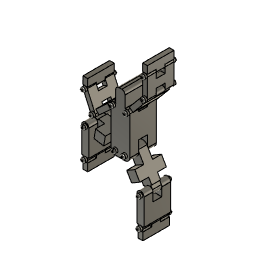
climber v7 (Autodesk Fusion 360 design; units mm, degrees)
Autodesk Fusion 360 part; units mm, degrees
sketch "Sketch1" plane through (0, 0, 0) normal (0, 1, 0) x (1, 0, 0) in component "climberTorso&Head"
  line L0 (1.4167, 0) -> (4.25, 0)
  line L1 (5.6667, -1.4167) -> (5.6667, -12.8917)
  line L2 (4.9583, -13.6) -> (0.7083, -13.6)
  line L3 (0, -12.8917) -> (0, -1.4167)
  circle A0 centre (0.7083, -12.8917) radius 0.25
  circle A1 centre (4.9583, -12.8917) radius 0.25
  circle A2 centre (1.4167, -1.4167) radius 0.25
  circle A3 centre (4.25, -1.4167) radius 0.25
  line L4 (1.4167, -13.6) -> (4.25, -13.6)
  line L5 (4.25, -13.6) -> (4.25, -17.1333)
  line L6 (3.25, -18.1333) -> (2.4167, -18.1333)
  line L7 (1.4167, -17.1333) -> (1.4167, -13.6)
  arc A4 (1.4167, -17.1333) -> (2.4167, -18.1333) centre (2.4167, -17.1333) ccw
  arc A5 (3.25, -18.1333) -> (4.25, -17.1333) centre (3.25, -17.1333) ccw
  line L8 (4.9583, -12.8917) -> (0.7083, -12.8917) construction
  line L9 (1.4167, -13.6) -> (1.4167, -12.8917) construction
  line L10 (1.4167, -12.8917) -> (1.4167, -13.6)
  line L11 (4.25, -12.8917) -> (4.25, -13.6)
  line L12 (4.9583, -12.1833) -> (5.6667, -12.1833)
  arc A6 (4.9583, -13.6) -> (5.6667, -12.8917) centre (4.9583, -12.8917) ccw
  arc A7 (4.9583, -12.1833) -> (4.25, -12.8917) centre (4.9583, -12.8917) ccw
  arc A8 (1.4167, -12.8917) -> (1.2092, -12.3908) centre (0.7083, -12.8917) ccw
  arc A9 (0, -12.8917) -> (0.7083, -13.6) centre (0.7083, -12.8917) ccw
  line L13 (0.7083, -12.8917) -> (0.7083, -12.1833) construction
  line L14 (4.9583, -12.8917) -> (4.9583, -12.1833) construction
  line L15 (4.25, -1.4167) -> (4.25, -2.8333) construction
  line L16 (1.4167, -1.4167) -> (1.4167, -2.8333) construction
  line L17 (1.4167, -2.8333) -> (0, -2.8333) construction
  line L18 (1.4167, -2.8333) -> (0, -2.8333)
  arc A10 (5.6667, -1.4167) -> (4.25, 0) centre (4.25, -1.4167) ccw
  arc A11 (2.8333, -1.4167) -> (3.2483, -2.4184) centre (4.25, -1.4167) ccw
  arc A12 (1.4167, 0) -> (0, -1.4167) centre (1.4167, -1.4167) ccw
  arc A13 (2.4184, -2.4184) -> (2.8333, -1.4167) centre (1.4167, -1.4167) ccw
  line L19 (1.2092, -12.3908) -> (0, -11.1816)
  line L20 (0.7083, -12.8917) -> (1.2092, -12.3908) construction
  line L21 (1.2092, -12.3908) -> (0, -11.1816)
  line L22 (1.2092, -12.3908) -> (0, -11.1816)
  circle A14 centre (1.4167, -1.4167) radius 1.4167 construction
  circle A15 centre (4.25, -1.4167) radius 1.4167 construction
  line L23 (1.4167, -1.4167) -> (2.4184, -2.4184) construction
  line L24 (4.25, -1.4167) -> (3.2483, -2.4184) construction
  line L25 (3.2483, -2.4184) -> (5.6667, -4.8368) construction
  line L26 (2.4184, -2.4184) -> (0, -4.8368) construction
  line L27 (3.2483, -2.4184) -> (5.6667, -4.8368)
  line L28 (2.4184, -2.4184) -> (0, -4.8368)
  point P0 (5.6667, 0)
  point P1 (0, -13.6)
  point P2 (1.4167, -18.1333)
  dimension "d69" = 5.6667
  dimension "d70" = 13.6
  dimension "d71" = 0.5
  dimension "d73" = 0.7083
  dimension "d75" = 0.7083
  dimension "d88" = 2.8333
  dimension "d89" = 4.5333
  dimension "d90" = 1
  dimension "d91" = 1
  dimension "d118" = 0.7083
  dimension "d145" = 1.4167
  dimension "d146" = 1.4167
  dimension "d149" = 0.7083
  dimension "d151" = 0.7083
  dimension "d152" = 0.7083
  dimension "d303" = 1.4167
  dimension "d304" = 1.4167
  dimension "d305" = 1.4167
  dimension "d306" = 2.8333
  dimension "d307" = 2.8333
  dimension "d308" = 1.4167
  dimension "d358" = 90
  constraint horizontal L0
  constraint vertical L1
  constraint horizontal L2
  constraint vertical L3
  constraint equal A1 A3
  constraint equal A0 A1
  constraint equal A0 A2
  constraint horizontal A2.centre A3.centre
  constraint horizontal A0.centre A1.centre
  constraint coincident P1 L2
  constraint coincident P1 L3
  constraint coincident origin L0
  constraint coincident origin L3
  constraint coincident P0 L0
  constraint coincident P0 L1
  constraint horizontal L4
  constraint vertical L5
  constraint horizontal L6
  constraint vertical L7
  constraint coincident P2 L6
  constraint coincident P2 L7
  constraint tangent L6 A4
  constraint tangent L7 A4
  constraint tangent L5 A5
  constraint tangent L6 A5
  constraint concentric A0 A8
  constraint coincident L3.start A8
  constraint concentric A1 A6
  constraint coincident A1.centre L8.start
  constraint coincident A0.centre L8.end
  constraint coincident L8 L9.end
  constraint tangent L9 A8
  constraint perpendicular L4 L10
  constraint coincident L8 L11.start
  constraint perpendicular L2 L11
  constraint coincident L12.start A6
  constraint perpendicular L1 L12
  constraint concentric A6 A7
  constraint concentric A8 A9
  constraint perpendicular L12 L14
  constraint concentric A2 A12
  constraint concentric A3 A10
  constraint coincident A3.centre L15.start
  constraint vertical L15
  constraint coincident A2.centre L16.start
  constraint coincident L16.end A12
  constraint vertical L16
  constraint coincident L3 L17.end
  constraint tangent L17 A12
  constraint perpendicular L3 L18
  constraint concentric A10 A11
  constraint concentric A12 A13
  constraint coincident L3 L19.end
  constraint perpendicular L19 L20
  constraint concentric A13 A14
  constraint concentric A10 A15
  constraint perpendicular L23 L24
  constraint coincident L1 L25.end
  constraint tangent A11 L25
  constraint perpendicular L24 L25
  constraint coincident L3 L26.end
  constraint tangent A15 L27
  measures "d69" distance of origin P0
  measures "d70" distance of origin P1
  measures "d71" diameter of A0
  measures "d73" distance of L2 A0.centre
  measures "d75" distance of L1 A1.centre
  measures "d88" distance of L4.start L4.end
  measures "d89" distance of L4.start P2
  measures "d90" radius of A4
  measures "d91" radius of A5
  measures "d118" distance of L3 A0.centre
  measures "d145" diameter of A8
  measures "d146" diameter of A6
  measures "d149" distance of L9.end L4.start
  measures "d151" distance of L11.start L4.end
  measures "d152" distance of L12.start L12.end
  measures "d303" distance of L3 A2.centre
  measures "d304" distance of L1 A3.centre
  measures "d305" distance of L0 A3.centre
  measures "d306" diameter of A12
  measures "d307" diameter of A10
  measures "d308" distance of L16.end L17.end
  measures "d358" angle of L25 L26
extrude "Extrude2" add sketch "Sketch1" along normal mid plane 8 makes body 1 in component "climberTorso&Head"
sketch "Sketch2" plane through (0, 0, 0) normal (0, 1, 0) x (1, 0, 0) in component "climberUpperArms"
  line L0 (1.4167, 2.1237) -> (1.4167, -6.0929)
  line L1 (0, -6.0929) -> (0, 2.1237)
  circle A0 centre (0.7083, -6.0929) radius 0.25
  circle A1 centre (0.7083, 2.1237) radius 0.25
  circle A2 centre (0.7083, -6.0929) radius 0.7083
  circle A3 centre (0.7083, 2.1237) radius 0.7083
  line L2 (0.7083, -6.0929) -> (0.7083, 2.1237) construction
  line L3 (0.7083, -5.3846) -> (0, -5.3846) construction
  line L4 (0.7083, -6.8013) -> (0.7083, 2.8321) construction
  line L5 (0.7083, -6.0929) -> (1.2092, -5.5921) construction
  line L6 (0.7083, -6.0929) -> (1.4167, -6.0929) construction
  line L7 (0.7083, -5.3846) -> (1.7101, -5.3846) construction
  line L8 (1.2092, -5.5921) -> (0, -4.3829) construction
  line L9 (1.2092, -5.5921) -> (-0.5009, -5.5921) construction
  line L10 (0, -4.3829) -> (1.4167, -4.3829)
  line L11 (0.7083, 2.1237) -> (1.2092, 1.6229) construction
  line L12 (0.7083, 2.1237) -> (1.4167, 2.1237) construction
  line L13 (1.2092, 1.6229) -> (0, 0.4137) construction
  line L14 (1.2092, 1.6229) -> (2.9193, 1.6229) construction
  line L15 (0, 0.4137) -> (1.4167, 0.4137)
  dimension "d106" = 0.5
  dimension "d108" = 0.7083
  dimension "d119" = 1.4167
  dimension "d120" = 1.4167
  dimension "d121" = 1.4167
  dimension "d132" = 0.7083
  dimension "d336" = 9.6333
  dimension "d341" = 45
  dimension "d342" = 0.7083
  dimension "d344" = 45
  dimension "d480" = 45
  dimension "d481" = 135
  constraint vertical L0
  constraint vertical L1
  constraint equal A0 A1
  constraint vertical A0.centre A1.centre
  constraint concentric A0 A2
  constraint concentric A1 A3
  constraint coincident A3 L1.end
  constraint coincident A3 L0.start
  constraint coincident A2 L1.start
  constraint coincident A2 L0.end
  constraint coincident A0.centre A2.centre
  constraint coincident A1.centre A3.centre
  constraint coincident L2 L3.start
  constraint coincident A2 L3.start
  constraint perpendicular L1 L3
  constraint coincident A2 L4.start
  constraint coincident A3 L4.end
  constraint horizontal L6
  constraint horizontal L7
  constraint horizontal L9
  constraint coincident L1 L8.end
  constraint coincident L0 L10.end
  constraint perpendicular L0 L10
  constraint horizontal L12
  constraint coincident A3 L11.end
  constraint horizontal L14
  constraint coincident L1 L13.end
  constraint coincident L0 L15.end
  constraint perpendicular L0 L15
  measures "d106" diameter of A0
  measures "d108" distance of L1 A0.centre
  measures "d119" diameter of A2
  measures "d120" diameter of A3
  measures "d121" distance of L0 L1
  measures "d132" distance of L3.start L3.end
  measures "d336" distance of L4.start L4.end
  measures "d341" angle of L5 L6
  measures "d342" distance of A0.centre L5.end
  measures "d344" angle of L8 L9
  measures "d480" angle of L11 L12
  measures "d481" angle of L13 L14
extrude "Extrude3" add sketch "Sketch2" along normal mid plane 2.6667 separate body contours A3 | L0 L1 A3 L15 | L0 L1 A2 L10 | A2 makes body 2 at (1.4158, 0.4444, 6.1282) makes body 3 at (0.1657, -0.4444, -2.579) in component "climberUpperArms"
extrude "Extrude2'" add sketch "Sketch2" along normal mid plane 8 separate body contours L0 L1 L10 L15 makes body 4 in component "climberUpperArms"
extrude "Extrude3'" cut sketch "Sketch1" along normal mid plane 2.6667 contours L0 L1 L3 A10 A11 A12 A13 L27 L28 | L1 L2 L11 L12 A6 A7 | L2 L3 L10 A8 A9 L19 L21 L22 | A0 | A1 | A2 | A3 bodies 1 in component "climberTorso&Head"
sketch "Sketch1 (2)" plane through (0, 0, 0) normal (0, 1, 0) x (1, 0, 0) in component "climberLowerArms"
  line L0 (3.9167, -0.375) -> (3.9167, -6.325)
  line L1 (2.5, -6.325) -> (2.5, -0.375)
  circle A0 centre (3.2083, -6.325) radius 0.25
  circle A1 centre (3.2083, -0.375) radius 0.25
  line L2 (3.2083, -6.325) -> (3.2083, -0.375) construction
  arc A2 (2.5, -6.325) -> (3.9167, -6.325) centre (3.2083, -6.325) ccw
  arc A3 (3.9167, -0.375) -> (2.5, -0.375) centre (3.2083, -0.375) ccw
  line L3 (3.2083, -6.325) -> (3.2083, -7.0333) construction
  line L4 (3.2083, -0.375) -> (3.2083, 0.3333) construction
  circle A4 centre (3.2083, -6.325) radius 0.7083 construction
  circle A5 centre (3.2083, -0.375) radius 0.7083 construction
  line L5 (3.2083, -6.325) -> (3.7092, -5.8241) construction
  line L6 (3.2083, -6.325) -> (3.9167, -6.325) construction
  line L7 (3.7092, -5.8241) -> (2.5, -4.6149) construction
  line L8 (2.5, -4.6149) -> (3.9167, -4.6149)
  line L9 (3.2083, -0.375) -> (3.7092, -0.8759) construction
  line L10 (3.2083, -0.375) -> (3.9167, -0.375) construction
  line L11 (3.7092, -0.8759) -> (2.5, -2.0851) construction
  line L12 (2.5, -2.0851) -> (3.9167, -2.0851)
  dimension "d186" = 0.5
  dimension "d188" = 0.7083
  dimension "d191" = 1.4167
  dimension "d192" = 1.4167
  dimension "d200" = 1.4167
  dimension "d201" = 7.3667
  dimension "d267" = 0
  dimension "d268" = 0
  dimension "d269" = 0
  dimension "d270" = 0
  dimension "d337" = 1.4167
  dimension "d338" = 1.4167
  dimension "d482" = 45
  dimension "d483" = 90
  dimension "d484" = 45
  dimension "d485" = 45
  dimension "d486" = 90
  dimension "d487" = 45
  constraint vertical L0
  constraint vertical L1
  constraint equal A0 A1
  constraint vertical A0.centre A1.centre
  constraint concentric A0 A2
  constraint concentric A1 A3
  constraint coincident A0.centre L2.start
  constraint coincident A1.centre L2.end
  constraint midpoint A2 L3.end
  constraint parallel L2 L3
  constraint midpoint A3 L4.end
  constraint parallel L2 L4
  constraint concentric A0 A4
  constraint concentric A1 A5
  constraint horizontal L6
  constraint coincident A4 L5.end
  constraint coincident L1 L7.end
  constraint coincident L0 L8.end
  constraint horizontal L10
  constraint coincident A5 L9.end
  constraint coincident L1 L11.end
  constraint coincident L0 L12.end
  measures "d186" diameter of A0
  measures "d188" distance of L1 A0.centre
  measures "d191" diameter of A2
  measures "d192" diameter of A3
  measures "d200" distance of L0 L1
  measures "d201" distance of L3.end L4.end
  measures "d337" diameter of A4
  measures "d338" diameter of A5
  measures "d482" angle of L5 L6
  measures "d483" angle of L5 L7
  measures "d484" angle of L7 L8
  measures "d485" angle of L9 L10
  measures "d486" angle of L9 L11
  measures "d487" angle of L11 L12
extrude "Extrude1" add sketch "Sketch1 (2)" along normal mid plane 8 separate body makes body 5 in component "climberLowerArms"
extrude "Extrude2''" cut sketch "Sketch1 (2)" along normal mid plane 2.6667 contours L0 L1 A3 L12 | L0 L1 A2 L8 | A0 bodies 5 in component "climberLowerArms"
sketch "Sketch1 (3)" plane through (0, 0, 0) normal (0, 1, 0) x (1, 0, 0) in component "climberHand"
  line L0 (3.9167, -1.7917) -> (3.9167, -4.7667)
  line L1 (3.9167, -4.7667) -> (2.5, -4.7667)
  line L2 (2.5, -4.7667) -> (2.5, -1.7917)
  circle A0 centre (3.2083, -1.7917) radius 0.25
  line L3 (3.2083, -1.7917) -> (3.2083, -4.7667) construction
  arc A1 (3.9167, -1.7917) -> (2.5, -1.7917) centre (3.2083, -1.7917) ccw
  line L4 (3.2083, -1.7917) -> (3.2083, -1.0833) construction
  circle A2 centre (3.2083, -1.7917) radius 0.7083 construction
  line L5 (3.2083, -2.5) -> (3.9167, -2.5) construction
  line L6 (3.9167, -2.5) -> (2.5, -2.5)
  dimension "d236" = 1.4167
  dimension "d237" = 0.5
  dimension "d239" = 0.7083
  dimension "d242" = 1.4167
  dimension "d245" = 3.6833
  dimension "d263" = 0
  dimension "d264" = 0
  dimension "d265" = 0
  dimension "d266" = 0
  dimension "d340" = 1.4167
  constraint vertical L0
  constraint horizontal L1
  constraint vertical L2
  constraint concentric A0 A1
  constraint coincident A0.centre L3.start
  constraint midpoint L1 L3.end
  constraint midpoint A1 L4.end
  constraint parallel L3 L4
  constraint coincident L4.end A2
  constraint coincident A2 L5.start
  constraint coincident L3 L5.start
  constraint coincident L0 L5.end
  constraint tangent A2 L5
  constraint perpendicular L0 L6
  measures "d236" distance of L0 L2
  measures "d237" diameter of A0
  measures "d239" distance of L2 A0.centre
  measures "d242" diameter of A1
  measures "d245" distance of L3.end L4.end
  measures "d340" distance of L5.end L6.end
extrude "Extrude1'" add sketch "Sketch1 (3)" along normal mid plane 8 separate body contours L0 L1 L2 L6 makes body 6 in component "climberHand"
extrude "Extrude2'''" add sketch "Sketch1 (3)" along normal mid plane 2.6667 bodies 6 in component "climberHand"
sketch "Sketch1 (4)" plane through (0, 0, 0) normal (0, 1, 0) x (1, 0, 0) in component "climberUpperLeg"
  line L0 (5.9167, -0.1667) -> (5.9167, -8.3833)
  line L1 (3.0833, -8.3833) -> (3.0833, -0.1667)
  circle A0 centre (4.5, -8.3833) radius 0.25
  circle A1 centre (4.5, 0.8958) radius 0.25
  line L2 (4.5, -9.8) -> (4.5, 1.9583) construction
  line L3 (4.5, -6.9667) -> (5.9167, -6.9667) construction
  line L4 (4.5, -5.8333) -> (5.9167, -5.8333) construction
  arc A2 (3.0833, -8.3833) -> (5.9167, -8.3833) centre (4.5, -8.3833) ccw
  circle A3 centre (4.5, -8.3833) radius 1.4167 construction
  line L5 (4.5, -8.3833) -> (5.5017, -7.3816) construction
  line L6 (4.5, -8.3833) -> (5.9167, -8.3833) construction
  line L7 (5.5017, -7.3816) -> (3.0833, -4.9632) construction
  line L8 (3.0833, -4.9632) -> (5.9167, -4.9632)
  line L9 (4.5, 2.6668) -> (4.5, 1.9583)
  line L10 (4.5, 0.8958) -> (5.5625, 0.8958) construction
  line L11 (4.5, 0.8958) -> (3.4375, 0.8958) construction
  line L12 (5.2083, 1.25) -> (5.2083, 1.25) construction
  line L13 (5.2083, 1.25) -> (5.2083, 1.25)
  line L14 (5.5625, 0.8958) -> (5.5625, -0.1667)
  line L15 (3.4375, 0.8958) -> (3.4375, -0.1667)
  arc A4 (5.5625, 0.8958) -> (3.4375, 0.8958) centre (4.5, 0.8958) ccw
  circle A5 centre (4.5, 0.8958) radius 1.0625 construction
  line L16 (4.5, 0.8958) -> (5.2513, 0.1445) construction
  line L17 (4.5, 0.8958) -> (5.5625, 0.8958) construction
  line L18 (5.2513, 0.1445) -> (3.0833, -2.0234) construction
  line L19 (3.0833, -2.0234) -> (5.9167, -2.0234)
  line L20 (3.4375, -0.1667) -> (3.0833, -0.1667)
  line L21 (5.5625, -0.1667) -> (5.9167, -0.1667) construction
  line L22 (5.9167, -0.1667) -> (5.5625, -0.1667)
  dimension "d285" = 0.5
  dimension "d287" = 1.4167
  dimension "d290" = 2.8333
  dimension "d292" = 1.4167
  dimension "d293" = 1.4167
  dimension "d296" = 11.7583
  dimension "d297" = 2.8333
  dimension "d359" = 45
  dimension "d381" = 0
  dimension "d382" = 0
  dimension "d383" = 0
  dimension "d384" = 0
  dimension "d393" = 0
  dimension "d394" = 0
  dimension "d395" = 0
  dimension "d396" = 0
  dimension "d411" = 1.0625
  dimension "d422" = 2.125
  dimension "d424" = 2.8333
  dimension "d488" = 45
  dimension "d489" = 90
  dimension "d490" = 45
  constraint vertical L0
  constraint vertical L1
  constraint equal A0 A1
  constraint vertical A0.centre A1.centre
  constraint concentric A0 A2
  constraint coincident L2 L3.start
  constraint perpendicular L2 L3
  constraint coincident L2 L4.start
  constraint coincident L0 L4.end
  constraint midpoint L2.start A2
  constraint concentric A0 A3
  constraint horizontal L6
  constraint coincident A0.centre A2.centre
  constraint coincident A3 L5.end
  constraint coincident L1 L7.end
  constraint perpendicular L5 L7
  constraint coincident L0 L8.end
  constraint perpendicular L0 L8
  constraint vertical L9
  constraint perpendicular L2 L10
  constraint perpendicular L2 L11
  constraint coincident A1.centre L10.start
  constraint perpendicular L2 L22
  constraint vertical L14
  constraint vertical L15
  constraint coincident L15.end L22
  constraint tangent L15 A4
  constraint concentric A1 A4
  constraint concentric A4 A5
  constraint horizontal L17
  constraint coincident A5 L16.end
  constraint coincident L1 L18.end
  constraint collinear L20 L22
  measures "d285" diameter of A0
  measures "d287" distance of L1 A0.centre
  measures "d290" diameter of A2
  measures "d292" distance of L3.start L3.end
  measures "d293" distance of L4.start L4.end
  measures "d296" distance of L2.start L2.end
  measures "d297" distance of L0 L1
  measures "d359" angle of L5 L6
  measures "d411" distance of A1.centre L2.end
  measures "d422" diameter of A4
  measures "d424" distance of L0.start L1.end
  measures "d488" angle of L16 L17
  measures "d489" angle of L16 L18
  measures "d490" angle of L18 L19
extrude "Extrude1''" add sketch "Sketch1 (4)" along normal mid plane 8 separate body contours L0 L1 L8 L19 makes body 7 in component "climberUpperLeg"
extrude "Extrude2''''" add sketch "Sketch1 (4)" along normal mid plane 2.6667 bodies 7 in component "climberUpperLeg"
sketch "Sketch1 (5)" plane through (0, 0, 0) normal (0, 1, 0) x (1, 0, 0) in component "climberLowerLeg"
  line L0 (-3.2308, -3.0625) -> (-3.2308, -10.925)
  line L1 (-5.3558, -10.925) -> (-5.3558, -3.0625)
  circle A0 centre (-4.2933, -10.925) radius 0.25
  circle A1 centre (-4.2933, -2.3542) radius 0.25
  line L2 (-4.2933, -10.925) -> (-4.2933, -11.9875) construction
  line L3 (-4.2933, -11.9875) -> (-4.2933, -1.6458) construction
  arc A2 (-5.3558, -10.925) -> (-3.2308, -10.925) centre (-4.2933, -10.925) ccw
  line L4 (-3.2308, -3.0625) -> (-3.2308, -1.6458) construction
  line L5 (-3.2308, -1.6458) -> (-4.2933, -1.6458) construction
  line L6 (-5.3558, -3.0625) -> (-5.3558, -1.6458) construction
  line L7 (-5.3558, -1.6458) -> (-4.2933, -1.6458) construction
  circle A3 centre (-4.2933, -2.3542) radius 0.7083 construction
  line L8 (-4.2933, -3.0625) -> (-3.2308, -3.0625) construction
  line L9 (-3.2308, -3.0625) -> (-5.3558, -3.0625)
  line L10 (-4.2933, -2.3542) -> (-3.585, -2.3542) construction
  line L11 (-4.2933, -2.3542) -> (-5.0017, -2.3542) construction
  line L12 (-3.585, -2.3542) -> (-3.585, -3.0625)
  line L13 (-5.0017, -2.3542) -> (-5.0017, -3.0625)
  arc A4 (-3.585, -2.3542) -> (-5.0017, -2.3542) centre (-4.2933, -2.3542) ccw
  circle A5 centre (-4.2933, -10.925) radius 1.0625 construction
  line L14 (-4.2933, -10.925) -> (-3.542, -10.1737) construction
  line L15 (-4.2933, -10.925) -> (-3.2308, -10.925) construction
  line L16 (-3.542, -10.1737) -> (-5.3558, -8.3599) construction
  line L17 (-5.3558, -8.3599) -> (-3.2308, -8.3599)
  dimension "d362" = 0.5
  dimension "d364" = 1.0625
  dimension "d368" = 2.125
  dimension "d369" = 10.3417
  dimension "d370" = 2.125
  dimension "d377" = 0
  dimension "d378" = 0
  dimension "d379" = 0
  dimension "d380" = 0
  dimension "d389" = 0
  dimension "d390" = 0
  dimension "d391" = 0
  dimension "d392" = 0
  dimension "d450" = 0.7083
  dimension "d451" = 1.4167
  dimension "d452" = 1.4167
  dimension "d453" = 90
  dimension "d454" = 180
  dimension "d455" = 0.7083
  dimension "d517" = 45
  dimension "d518" = 90
  dimension "d519" = 45
  constraint vertical L0
  constraint vertical L1
  constraint equal A0 A1
  constraint vertical A0.centre A1.centre
  constraint concentric A0 A2
  constraint coincident A0.centre L2.start
  constraint coincident L2.end A2
  constraint vertical L2
  constraint parallel L2 L3
  constraint vertical L4
  constraint vertical L6
  constraint concentric A1 A3
  constraint concentric A1 A4
  constraint horizontal L8
  constraint coincident A3 L8.start
  constraint coincident L3 L8.start
  constraint perpendicular L1 L9
  constraint coincident A1.centre A3.centre
  constraint coincident A3 L10.end
  constraint perpendicular L3 L10
  constraint parallel L10 L11
  constraint coincident L9 L12.end
  constraint coincident L1.end L6.start
  constraint coincident L0.start L4.start
  constraint concentric A2 A5
  constraint horizontal L15
  constraint coincident A5 L14.end
  constraint coincident L1 L16.end
  constraint coincident L0 L17.end
  measures "d362" diameter of A0
  measures "d364" distance of L1 A0.centre
  measures "d368" diameter of A2
  measures "d369" distance of L2.end L3.end
  measures "d370" distance of L0 L1
  measures "d450" distance of A1.centre L7
  measures "d451" diameter of A3
  measures "d452" diameter of A4
  measures "d453" angle of L11 L12
  measures "d454" angle of L12 L13
  measures "d455" distance of L11.end L13.end
  measures "d517" angle of L14 L15
  measures "d518" angle of L14 L16
  measures "d519" angle of L16 L17
extrude "Extrude1'''" add sketch "Sketch1 (5)" along normal mid plane 8 separate body makes body 8 in component "climberLowerLeg"
extrude "Extrude2'''''" cut sketch "Sketch1 (5)" along normal mid plane 2.6667 contours L0 L1 A2 L17 | L9 L12 L13 A4 | A0 bodies 8 in component "climberLowerLeg"
sketch "Sketch1 (6)" plane through (0, 0, 0) normal (0, 1, 0) x (1, 0, 0) in component "climberFoot"
  line L0 (-10, -5) -> (-8.5833, -5)
  line L1 (-8.5833, -5) -> (-8.5833, -7.975)
  line L2 (-10, -7.975) -> (-10, -5)
  circle A0 centre (-9.2917, -7.975) radius 0.25
  line L3 (-9.2917, -7.975) -> (-9.2917, -8.6833) construction
  line L4 (-9.2917, -7.975) -> (-9.2917, -5) construction
  line L5 (-9.2917, -7.2667) -> (-8.5833, -7.2667) construction
  line L6 (-8.5833, -7.2667) -> (-10, -7.2667)
  arc A1 (-10, -7.975) -> (-8.5833, -7.975) centre (-9.2917, -7.975) ccw
  dimension "d437" = 1.4167
  dimension "d439" = 0.5
  dimension "d441" = 0.7083
  dimension "d443" = 1.4167
  dimension "d444" = 90
  dimension "d445" = 3.6833
  constraint horizontal L0
  constraint vertical L1
  constraint vertical L2
  constraint concentric A0 A1
  constraint vertical L3
  constraint coincident A0.centre L3.start
  constraint coincident L3.end A1
  constraint midpoint L0 L4.end
  constraint coincident L4 L5.start
  constraint coincident L1 L5.end
  constraint coincident L2 L6.end
  constraint perpendicular L2 L6
  measures "d437" distance of L0.start L0.end
  measures "d439" diameter of A0
  measures "d441" distance of L2 A0.centre
  measures "d443" diameter of A1
  measures "d444" angle of L4 L5
  measures "d445" distance of L3.end L4.end
extrude "Extrude1''''" add sketch "Sketch1 (6)" along normal mid plane 8 separate body contours L0 L1 L2 L6 makes body 9 in component "climberFoot"
extrude "Extrude2''''''" add sketch "Sketch1 (6)" along normal mid plane 2.6667 contours L1 L2 L6 A1 bodies 9 in component "climberFoot"
sketch "Sketch1 (7)" plane through (0, 0, 0) normal (0, 1, 0) x (1, 0, 0) in component "jointPin"
  circle A0 centre (5, -6) radius 0.225
  dimension "d520" = 0.45
  measures "d520" diameter of A0
extrude "Extrude1'''''" add sketch "Sketch1 (7)" along normal mid plane 10 separate body makes body 10 in component "jointPin"
sketch "Sketch3" plane through (0, -5, 0) normal (0, -1, 0) x (1, 0, 0) in component "jointPin"
  circle A0 centre (5, 6) radius 0.225
  circle A1 centre (5, 6) radius 0.675
  dimension "d526" = 1.35
  constraint concentric A0 A1
  measures "d526" diameter of A1
extrude "Extrude2'''''''" add sketch "Sketch3" against normal blind 1 separate body contours A0 | A1 makes body 11 in component "jointPin"
sketch "Sketch4" plane through (0, 5, 0) normal (0, 1, 0) x (-1, 0, 0) in component "jointPin"
  circle A0 centre (-5, 6) radius 0.225
  circle A1 centre (-5, 6) radius 0.675
  dimension "d531" = 1.35
  constraint concentric A0 A1
  measures "d531" diameter of A1
extrude "Extrude3''" add sketch "Sketch4" against normal blind 1 separate body contours A0 | A1 makes body 12 in component "jointPin"
fillet "Fillet3" radius 0.45 curvature continuous 1 edges at (4.3707, -5, 5.7559) on bodies 11 in component "jointPin"
fillet "Fillet4" radius 0.4 curvature continuous 1 edges at (5.6293, 5, 5.7559) on bodies 12 in component "jointPin"
component "climberTorso&Head" placed x (1, 0, 0) y (0, 1, 0) z (0, 0, 1) at (0, 0, 0)
component "climberUpperArms" placed x (-0.672784, 0, 0.739839) y (0, -1, 0) z (0.739839, 0, 0.672784) at (-3.3229, 0, 8.2684)
component "climberUpperArms" placed x (-0.766044, 0, 0.642788) y (0, 1, 0) z (-0.642788, 0, -0.766044) at (9.4174, 0, 17.1038)
component "climberLowerArms" placed x (-1, 0, 0) y (0, 1, 0) z (0, 0, -1) at (13.4482, 0, 25.511)
component "climberLowerArms" placed x (0.915787, 0, 0.401665) y (0, -1, 0) z (0.401665, 0, -0.915787) at (-10.8494, 0, 11.8673)
component "climberHand" placed x (-0.999822, 0, 0.018887) y (0, -1, 0) z (0.018887, 0, 0.999822) at (-4.5867, 0, 10.9606)
component "climberHand" placed x (1, 0, 0) y (0, 1, 0) z (0, 0, 1) at (7.0316, 0, 23.3443)
component "climberUpperLeg" placed x (0.866025, 0, 0.5) y (0, 1, 0) z (-0.5, 0, 0.866025) at (4.5446, 0, -8.0935)
component "climberUpperLeg" placed x (-0.173648, 0, -0.984808) y (0, 1, 0) z (0.984808, 0, -0.173648) at (-6.0579, 0, 7.3041)
component "climberLowerLeg" placed x (-1, 0, 0) y (0, -1, 0) z (0, 0, 1) at (-12.0149, 0, -7.897)
component "climberLowerLeg" placed x (-1, 0, 0) y (0, -1, 0) z (0, 0, 1) at (4.5963, 0, -17.5443)
component "climberFoot" placed x (-1, 0, 0) y (0, -1, 0) z (0, 0, 1) at (-17.0132, 0, -13.5179)
component "climberFoot" placed x (-1, 0, 0) y (0, -1, 0) z (0, 0, 1) at (-0.4021, 0, -23.1652)
component "jointPins" placed x (1, 0, 0) y (0, 1, 0) z (0, 0, 1) at (0, 0, 0)
component "jointPin" placed x (1, 0, 0) y (0, 1, 0) z (0, 0, 1) at (-0.0417, 0, 6.8917) in component "jointPins"
component "jointPin" placed x (1, 0, 0) y (0, 1, 0) z (0, 0, 1) at (-12.7215, 0, -11.5429) in component "jointPins"
component "jointPin" placed x (-0.173648, 0, -0.984808) y (0, 1, 0) z (0.984808, 0, -0.173648) at (-12.7621, 0, 8.9939) in component "jointPins"
component "jointPin" placed x (0.866025, 0, 0.5) y (0, 1, 0) z (-0.5, 0, 0.866025) at (7.5595, 0, -14.3155) in component "jointPins"
component "jointPin" placed x (0.766044, 0, -0.642788) y (0, 1, 0) z (0.642788, 0, 0.766044) at (2.553, 0, 17.8037) in component "jointPins"
component "jointPin" placed x (1, 0, 0) y (0, 1, 0) z (0, 0, 1) at (5.2399, 0, 19.136) in component "jointPins"
component "jointPin" placed x (0.810004, 0, 0.586424) y (0, 1, 0) z (-0.586424, 0, 0.810004) at (-5.9022, 0, -0.4285) in component "jointPins"
component "jointPin" placed x (0.866025, 0, 0.5) y (0, 1, 0) z (-0.5, 0, 0.866025) at (2.9199, 0, -6.2795) in component "jointPins"
component "jointPin" placed x (-0.173648, 0, -0.984808) y (0, 1, 0) z (0.984808, 0, -0.173648) at (-3.6239, 0, 7.3826) in component "jointPins"
component "jointPin" placed x (1, 0, 0) y (0, 1, 0) z (0, 0, 1) at (-4.2917, 0, 6.8917) in component "jointPins"
component "jointPin" placed x (1, 0, 0) y (0, 1, 0) z (0, 0, 1) at (3.8896, 0, -21.1902) in component "jointPins"
component "jointPin" placed x (0.999822, 0, -0.018887) y (0, 1, 0) z (0.018887, 0, 0.999822) at (-12.873, 0, 6.9081) in component "jointPins"
equation "climberHeight = 34 mm"
equation "climberHeadLength = climberHeight / 7.5"
equation "materialThickness = 8 mm"
equation "climberTorsoLength = climberHeadLength * 3"
equation "climberUpperLegLength = climberHeadLength * 1.5"
equation "climberLowerLegLength = climberHeadLength * 1.5"
equation "climberFootLength = climberHeadLength * 0.5"
equation "climberUpperArmLength = 1.5 * climberHeadLength"
equation "climberLowerArmLegnth = climberHeadLength"
equation "climberHandLength = 0.5 * climberHeadLength"
equation "climberHeadWidth = climberHeadLength / 1.6"
equation "climberTorsoWidth = 2 * climberHeadWidth"
equation "climberUpperArmWidth = climberHeadWidth * 0.5"
equation "climberUpperLegWidth = climberHeadWidth"
equation "climberLowerLegWidth = climberHeadWidth * 0.75"
equation "climberLowerArmWidth = climberHeadWidth * 0.5"
equation "climberHandWidth = climberHeadWidth * 0.5"
equation "climberFootWidth = climberHeadWidth * 0.5"
equation "jointHoleDiameter = 0.5 mm"
equation "jointHoleShoulder_distanceFromEdge = climberUpperArmWidth / 2"
equation "d69 = climberTorsoWidth"
equation "d70 = climberTorsoLength"
equation "d71 = jointHoleDiameter"
equation "d73 = jointHoleShoulder_distanceFromEdge"
equation "d75 = jointHoleShoulder_distanceFromEdge"
equation "climberHeadFilletDistance = 1 mm"
equation "d88 = climberHeadWidth"
equation "d89 = climberHeadLength"
equation "d90 = climberHeadFilletDistance"
equation "d91 = climberHeadFilletDistance"
equation "d106 = jointHoleDiameter"
equation "jointHoleUpperArm_distanceFromEdgeCO = climberUpperArmWidth / 2"
equation "d108 = jointHoleUpperArm_distanceFromEdgeCO"
equation "d116 = materialThickness"
equation "d118 = jointHoleShoulder_distanceFromEdge"
equation "d119 = climberUpperArmWidth"
equation "d120 = climberUpperArmWidth"
equation "d121 = climberUpperArmWidth"
equation "d132 = climberUpperArmWidth / 2"
equation "d141 = materialThickness"
equation "d143 = materialThickness / 3"
equation "d145 = jointHoleShoulder_distanceFromEdge * 2"
equation "d146 = jointHoleShoulder_distanceFromEdge * 2"
equation "d147 = materialThickness"
equation "d149 = jointHoleShoulder_distanceFromEdge"
equation "d151 = jointHoleShoulder_distanceFromEdge"
equation "d152 = jointHoleShoulder_distanceFromEdge"
equation "d157 = materialThickness / 3"
equation "d186 = jointHoleDiameter"
equation "jointHoleLowerArm_distanceToEdgeCO = climberLowerArmWidth / 2"
equation "d188 = jointHoleLowerArm_distanceToEdgeCO"
equation "d191 = climberLowerArmWidth"
equation "d192 = climberHandWidth"
equation "d200 = climberLowerArmWidth"
equation "d201 = climberLowerArmLegnth + climberLowerArmWidth + climberHandWidth"
equation "d202 = materialThickness"
equation "d204 = materialThickness / 3"
equation "d236 = climberHandWidth"
equation "d237 = jointHoleDiameter"
equation "jointHoleHand_distanceToEdgeCO = climberHandWidth / 2"
equation "d239 = jointHoleHand_distanceToEdgeCO"
equation "d242 = jointHoleHand_distanceToEdgeCO * 2"
equation "d245 = climberHandLength + climberHandWidth"
equation "d247 = materialThickness"
equation "d249 = materialThickness / 3"
equation "d285 = jointHoleDiameter"
equation "jointHoleUpperLeg_distanceToEdgeCO = climberUpperLegWidth / 2"
equation "d287 = jointHoleUpperLeg_distanceToEdgeCO"
equation "d290 = climberUpperLegWidth"
equation "d292 = climberUpperLegWidth / 2"
equation "d293 = climberUpperLegWidth / 2"
equation "d296 = climberUpperLegLength + climberUpperLegWidth + climberLowerLegWidth"
equation "d297 = climberUpperLegWidth"
equation "d298 = materialThickness"
equation "jointHoleHips_distanceToEdgeCO = climberUpperLegWidth / 2"
equation "d303 = jointHoleHips_distanceToEdgeCO"
equation "d304 = jointHoleHips_distanceToEdgeCO"
equation "d305 = jointHoleHips_distanceToEdgeCO"
equation "d306 = climberUpperLegWidth"
equation "d307 = climberUpperLegWidth"
equation "d308 = jointHoleHips_distanceToEdgeCO"
equation "d336 = climberUpperArmLength + 2 * climberUpperArmWidth"
equation "d337 = climberLowerArmWidth"
equation "d338 = climberLowerArmWidth"
equation "d340 = climberHandWidth"
equation "d362 = jointHoleDiameter"
equation "jointHoleLowerLeg_distanceToEdgeCO = climberLowerLegWidth / 2"
equation "d364 = jointHoleLowerLeg_distanceToEdgeCO"
equation "d368 = climberLowerLegWidth"
equation "d369 = climberLowerLegLength + climberLowerLegWidth + climberFootWidth"
equation "d370 = climberLowerLegWidth"
equation "d373 = materialThickness"
equation "d375 = materialThickness / 3"
equation "d411 = jointHoleLowerLeg_distanceToEdgeCO"
equation "d422 = climberLowerLegWidth"
equation "d424 = climberUpperLegWidth"
equation "d437 = climberFootWidth"
equation "d439 = jointHoleDiameter"
equation "jointHoleFoot_distanceToEdgeCO = climberFootWidth / 2"
equation "d441 = jointHoleFoot_distanceToEdgeCO"
equation "d443 = climberFootWidth"
equation "d445 = climberFootLength + climberFootWidth"
equation "d446 = materialThickness"
equation "d448 = materialThickness / 3"
equation "d450 = jointHoleFoot_distanceToEdgeCO"
equation "d451 = climberFootWidth"
equation "d452 = climberFootWidth"
equation "d520 = jointPinDiameter"
equation "d521 = jointPinLength"
equation "jointPinDiameter = 0.9 * jointHoleDiameter"
equation "jointPinCapDiameter = 3 * jointPinDiameter"
equation "jointPinLength = 1.25 * materialThickness"
equation "d526 = jointPinCapDiameter"
equation "jointPinCapThickness = 0.125 * materialThickness"
equation "d528 = -jointPinCapThickness"
equation "d531 = jointPinCapDiameter"
equation "d532 = -jointPinCapThickness"
equation "jointPinCapFilletDistance = 0.4 * jointPinCapThickness"
equation "d549 = jointPinCapFilletDistance"
